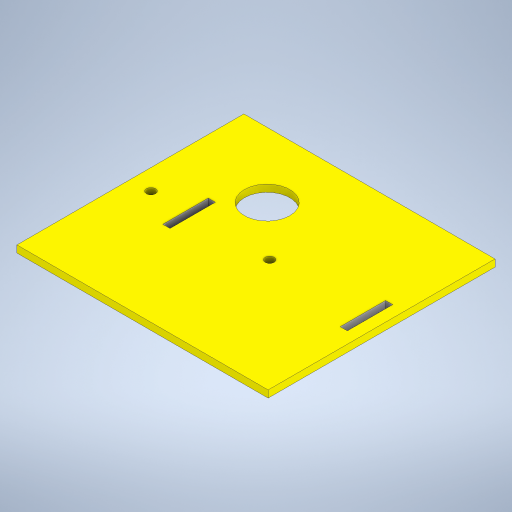
# Autodesk Inventor part: Base
Saved by Autodesk Inventor 2024 (Build 280153000, 153)
## iProperties
Created: 2024-04-22
Part Number: Base
Material: Generic
Document SubType Name: Modeling
Designer: samue
Density: 1 g/cm^3
Appearance: Default
Author: samue
Autodesk Inventor part; units mm, degrees
ref_plane "YZ Plane" through (0, 0, 0) normal (1, 0, 0) x (0, 1, 0)
ref_plane "XZ Plane" through (0, 0, 0) normal (0, 1, 0) x (-1, 0, 0)
ref_plane "XY Plane" through (0, 0, 0) normal (0, 0, 1) x (1, 0, 0)
sketch "Sketch1" plane through (0, 0, 0) normal (0, 1, 0) x (-1, 0, 0)
  line L0 (70, 50) -> (-70, 50)
  line L1 (-70, 50) -> (-70, -50)
  line L2 (-70, -50) -> (70, -50)
  line L3 (70, -50) -> (70, 50)
  line L4 (70, 50) -> (-70, -50) construction
  line L5 (-70, 50) -> (70, -50) construction
  point P0 (0, 0)
  dimension "d0" = 140
  dimension "d1" = 100
  constraints: 12 end point, 2 midpoint, 2 parallel, 1 horizontal, 1 perpendicular
  measures "d0" distance of L2.end L1.end
  measures "d1" distance of L0.end L1.end
extrude "Extrusion1" add sketch "Sketch1" along normal blind 3.125
sketch "Sketch9" plane through (0, 3.125, 0) normal (0, 1, 0) x (1, 0, 0)
  circle A0 centre (-1.7146, 21.2758) radius 10
  point P0 (0, 0)
  dimension "d41" = 20
  constraints: 1 centre point
  measures "d41" diameter of A0
extrude "Extrusion9" cut sketch "Sketch9" against normal blind 10
sketch "Sketch10" plane through (0, 3.125, 0) normal (0, 1, 0) x (1, 0, 0)
  circle A0 centre (-31.6428, 0) radius 2
  point P0 (0, 0)
  dimension "d44" = 4
  constraints: 1 centre point
  measures "d44" diameter of A0
extrude "Extrusion10" cut sketch "Sketch10" against normal blind 5
sketch "Sketch11" plane through (0, 3.125, 0) normal (0, 1, 0) x (1, 0, 0)
  circle A0 centre (20.6742, 0) radius 2
  point P0 (0, 0)
  dimension "d47" = 4
  constraints: 1 centre point
  measures "d47" diameter of A0
extrude "Extrusion11" cut sketch "Sketch11" against normal blind 5
sketch "Sketch15" plane through (0, 3.125, 0) normal (0, 1, 0) x (1, 0, 0)
  line L0 (-16.402, 10) -> (-13.247, 10)
  line L1 (-13.247, 10) -> (-13.247, -10)
  line L2 (-13.247, -10) -> (-16.402, -10)
  line L3 (-16.402, -10) -> (-16.402, 10)
  line L4 (-16.402, 10) -> (-13.247, -10) construction
  line L5 (-13.247, 10) -> (-16.402, -10) construction
  line L6 (61.753, 10) -> (64.908, 10)
  line L7 (64.908, 10) -> (64.908, -10)
  line L8 (64.908, -10) -> (61.753, -10)
  line L9 (61.753, -10) -> (61.753, 10)
  line L10 (61.753, 10) -> (64.908, -10) construction
  line L11 (64.908, 10) -> (61.753, -10) construction
  point P0 (0, 0)
  point P1 (-14.8245, 0)
  point P2 (63.3305, 0)
  dimension "d68" = 3.155
  dimension "d69" = 20
  dimension "d70" = 3.155
  dimension "d71" = 20
  dimension "d72" = 75
  constraints: 24 end point, 4 midpoint, 4 parallel, 2 horizontal, 2 perpendicular
  measures "d68" distance of L1.end L2.end
  measures "d69" distance of L0.end L1.end
  measures "d70" distance of L7.end L8.end
  measures "d71" distance of L6.end L7.end
  measures "d72" distance between parallel lines of L9 L1
extrude "Extrusion14" cut sketch "Sketch15" against normal blind 3.125
sketch "Sketch16" plane through (0, 3.125, 0) normal (0, 1, 0) x (1, 0, 0)
  line L0 (-70, -50) -> (70, -50) projected
  line L1 (-70, 50) -> (-40.7108, 50)
  line L2 (-40.7108, 50) -> (-40.7108, -50)
  line L3 (-40.7108, -50) -> (-70, -50)
  line L4 (-70, -50) -> (-70, 50)
  point P0 (0, 0)
  constraints: 8 end point, 2 parallel, 1 horizontal, 1 perpendicular, 1 point on line
extrude "Extrusion15" cut sketch "Sketch16" against normal blind 3.125
body "Solid1"
